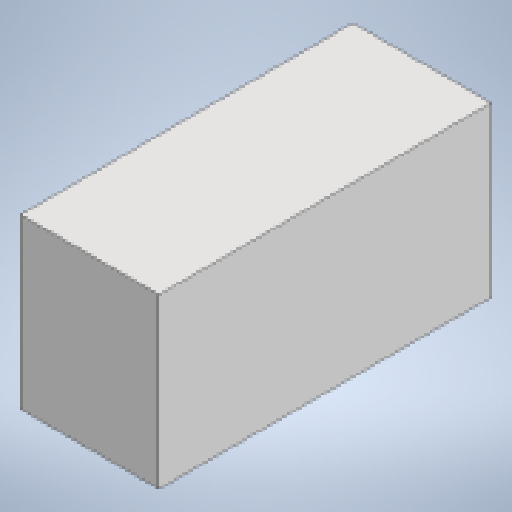
# Autodesk Inventor part: BK12_Spacer
Saved by Autodesk Inventor 2023 (Build 270158000, 158)
## iProperties
Created: 2022-05-01
Part Number: BK12_Spacer
Material: Generic
Document SubType Name: Modeling
Designer: plebbb
Density: 1 g/cm^3
Appearance: Default
Author: plebbb
Autodesk Inventor part; units mm, degrees
ref_plane "YZ Plane" through (0, 0, 0) normal (1, 0, 0) x (0, 1, 0)
ref_plane "XZ Plane" through (0, 0, 0) normal (0, 1, 0) x (-1, 0, 0)
ref_plane "XY Plane" through (0, 0, 0) normal (0, 0, 1) x (1, 0, 0)
sketch "Sketch1" plane through (0, 0, 0) normal (0, 1, 0) x (-1, 0, 0)
  line L0 (0, 0) -> (25, 0)
  line L1 (25, 0) -> (25, -60)
  line L2 (25, -60) -> (0, -60)
  line L3 (0, -60) -> (0, 0)
  circle A0 centre (19, -7) radius 3
  circle A1 centre (19, -53) radius 3
  circle A2 centre (6, -53) radius 3
  circle A3 centre (6, -7) radius 3
  line L4 (19, -7) -> (6, -7) construction
  line L5 (6, -7) -> (6, -53) construction
  line L6 (6, -53) -> (19, -53) construction
  line L7 (19, -53) -> (19, -7) construction
  point P0 (19, -30)
  point P1 (25, -30)
  point P2 (12.5, -53)
  point P3 (12.5, -60)
  dimension "d0" = 60
  dimension "d1" = 25
  dimension "d2" = 13
  dimension "d3" = 46
  dimension "d4" = 6
  constraints: 16 end point, 4 centre point, 4 midpoint, 4 parallel, 3 coincident, 3 equal radius, 2 horizontal, 2 perpendicular, 1 horizontal alignment, 1 vertical alignment
  measures "d0" distance of L0.end L1.end
  measures "d1" distance of L1.end L2.end
  measures "d2" distance of L5.end L6.end
  measures "d3" distance of L6.end L4.start
  measures "d4" diameter of A0
extrude "Extrusion1" add sketch "Sketch1" along normal blind 30.4
sketch "Sketch2" plane through (-25, 0, 0) normal (0, 0, 1) x (1, 0, 0)
  line L0 (0, 0) -> (25, 0) projected
  line L1 (25, 0) -> (25, 30.4) projected
  line L2 (0, 30.4) -> (25, 30.4) projected
  line L3 (0, 0) -> (0, 30.4) projected
extrude "Extrusion2" add sketch "Sketch2" along normal blind 2.917
body "Solid1"
